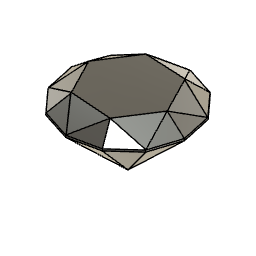
Rohini_diamond (Autodesk Fusion 360 design; units mm, degrees)
Autodesk Fusion 360 part; units mm, degrees
sketch "Sketch1" plane through (0, 0, 0) normal (0, 0, 1) x (1, 0, 0)
  line L0 (62.5, -82.5) -> (-62.5, -82.5)
  line L1 (-83.3163, -62.5) -> (-83.3163, 62.5)
  line L2 (-62.5, 82.5) -> (62.5, 82.5)
  line L3 (83.3163, 62.5) -> (83.3163, -62.5)
  line L4 (0, 82.5) -> (0, -82.5)
  line L5 (-83.3163, 0) -> (81.6837, 0)
  line L6 (-83.3163, 62.5) -> (-62.5, 82.5)
  line L7 (83.3163, 62.5) -> (62.5, 82.5)
  line L8 (83.3163, -62.5) -> (62.5, -82.5)
  line L9 (-83.3163, -62.5) -> (-62.5, -82.5)
  dimension "d1" = 165
  dimension "d2" = 165
  dimension "d3" = 125
  dimension "d4" = 125
  constraint horizontal L0
  constraint perpendicular L0 L1
  constraint parallel L0 L2
  constraint parallel L1 L3
  constraint perpendicular L1 L5
  constraint coincident L2 L4.start
  constraint coincident L1 L5.start
  constraint coincident L0 L4.end
  constraint midpoint origin L4
  measures "d1" distance of L5.start L5.end
  measures "d2" distance of L4.start L4.end
  measures "d3" distance of L3.start L3.end
  measures "d4" distance of L0.start L0.end
sketch "Sketch4" plane through (0, 0, 0) normal (0, 0, 1) x (1, 0, 0)
  line L0 (51.7018, -2.5335) -> (46.0418, 23.6568)
  line L1 (46.0418, 23.6568) -> (28.0449, 43.5083)
  line L2 (28.0449, 43.5083) -> (2.5335, 51.7018)
  line L3 (2.5335, 51.7018) -> (-23.6568, 46.0418)
  line L4 (-23.6568, 46.0418) -> (-43.5083, 28.0449)
  line L5 (-43.5083, 28.0449) -> (-51.7018, 2.5335)
  line L6 (-51.7018, 2.5335) -> (-46.0418, -23.6568)
  line L7 (-46.0418, -23.6568) -> (-28.0449, -43.5083)
  line L8 (-28.0449, -43.5083) -> (-2.5335, -51.7018)
  line L9 (-2.5335, -51.7018) -> (23.6568, -46.0418)
  line L10 (23.6568, -46.0418) -> (43.5083, -28.0449)
  line L11 (43.5083, -28.0449) -> (51.7018, -2.5335)
  dimension "d9" = 50
  measures "d9" distance of origin L11
extrude "Extrude2" add sketch "Sketch4" against normal blind 50 draft -45.5
extrude "Extrude3" add 1 faces at (5.7727, -11.235, 0) along direction (0, 0, 1) blind 1.5 draft -5
extrude "Extrude4" add 1 faces at (1.8817, -8.7072, 1.5) along direction (0, 0, 1) blind 12.5 draft -50.5
ref_plane "WorkPlane2" through (16.4202, -31.9577, 14) normal (-0.437388, 0.281935, -0.853934) x (-0.541787, -0.840516, 0)
sketch "Sketch5" plane through (16.4202, -31.9577, 14) normal (-0.437388, 0.281935, -0.853934) x (-0.541787, -0.840516, 0)
  line L0 (0, 0) -> (-18.0379, -23.8291)
  line L1 (-18.0379, -23.8291) -> (-36.1563, 0)
  line L2 (-36.1563, 0) -> (0, 0)
  constraint coincident L0.start L2.end
  constraint horizontal L2
extrude "Extrude5" cut sketch "Sketch5" against normal blind 17
ref_plane "WorkPlane3" through (35.8863, -1.7585, 14) normal (-0.462857, -0.237822, -0.853934) x (0.457015, -0.889459, 0)
sketch "Sketch6" plane through (35.8863, -1.7585, 14) normal (-0.462857, -0.237822, -0.853934) x (0.457015, -0.889459, 0)
  line L0 (0, 0) -> (-35, 0)
  line L1 (-35, 0) -> (-17.5, -24.4191)
  line L2 (-17.5, -24.4191) -> (0, 0)
  constraint coincident L0.start L2.end
  constraint horizontal L0
extrude "Extrude6" cut sketch "Sketch6" against normal blind 17
ref_plane "WorkPlane4" through (19.466, 30.1992, 14) normal (-0.025469, -0.519757, -0.853934) x (0.998802, -0.048943, 0)
sketch "Sketch7" plane through (19.466, 30.1992, 14) normal (-0.025469, -0.519757, -0.853934) x (0.998802, -0.048943, 0)
  line L0 (0, 0) -> (-35.8879, 0)
  line L1 (-35.8879, 0) -> (-17.9439, -23.5661)
  line L2 (-17.9439, -23.5661) -> (0, 0)
  constraint coincident L0.start L2.end
  constraint horizontal L0
extrude "Extrude7" cut sketch "Sketch7" against normal blind 17
ref_plane "WorkPlane5" through (-16.3694, 31.9686, 14) normal (0.436815, -0.282198, -0.854141) x (0.542645, 0.839962, 0)
sketch "Sketch8" plane through (-16.3694, 31.9686, 14) normal (0.436815, -0.282198, -0.854141) x (0.542645, 0.839962, 0)
  line L0 (0, 0) -> (-35, 0)
  line L1 (-35, 0) -> (-18.1169, -23.6508)
  line L2 (-18.1169, -23.6508) -> (0, 0)
  constraint coincident L0.start L2.end
  constraint horizontal L0
extrude "Extrude8" cut sketch "Sketch8" against normal blind 17
ref_plane "WorkPlane6" through (-35.8863, 1.7585, 14) normal (0.462857, 0.237822, -0.853934) x (-0.457015, 0.889459, 0)
sketch "Sketch9" plane through (-35.8863, 1.7585, 14) normal (0.462857, 0.237822, -0.853934) x (-0.457015, 0.889459, 0)
  line L0 (0, 0) -> (-35, 0)
  line L1 (-35, 0) -> (-17.5, -23.9577)
  line L2 (-17.5, -23.9577) -> (0, 0)
  constraint coincident L0.start L2.end
  constraint horizontal L0
extrude "Extrude9" cut sketch "Sketch9" against normal blind 17
ref_plane "WorkPlane7" through (16.4202, -31.9577, 14) normal (0.036501, 0.511872, -0.858286) x (-0.997467, 0.071128, 0)
sketch "Sketch10" plane through (16.4202, -31.9577, 14) normal (0.036501, 0.511872, -0.858286) x (-0.997467, 0.071128, 0)
  line L0 (36.8018, 0) -> (0, 0)
  line L1 (0, 0) -> (17.4531, -24.0672)
  line L2 (17.4531, -24.0672) -> (36.8018, 0)
  constraint coincident L0.end L1.start
  constraint horizontal L0
extrude "Extrude10" cut sketch "Sketch10" against normal blind 17
